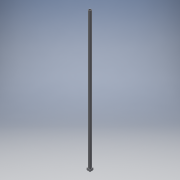
# Autodesk Inventor part: InnerLever
Saved by Autodesk Inventor 2017 (Build 210142000, 142)
## iProperties
Created: 2019-01-31
Part Number: InnerLever
Material: Generic
Document SubType Name: Modeling
Designer: S338674153
Density: 1 g/cm^3
Appearance: Default
Author: S338674153
Autodesk Inventor part; units mm, degrees
ref_plane "YZ Plane" through (0, 0, 0) normal (1, 0, 0) x (0, 1, 0)
ref_plane "XZ Plane" through (0, 0, 0) normal (0, 1, 0) x (-1, 0, 0)
ref_plane "XY Plane" through (0, 0, 0) normal (0, 0, 1) x (1, 0, 0)
sketch "Sketch1" plane through (0, 0, 0) normal (0, 1, 0) x (-1, 0, 0)
  circle A0 centre (0, 0) radius 6.985
  circle A1 centre (0, 0) radius 5.715
  dimension "d0" = 13.97
  dimension "d1" = 11.43
  constraints: 2 centre point, 2 coincident
  measures "d0" diameter of A0
  measures "d1" diameter of A1
extrude "Extrusion1" add sketch "Sketch1" along normal blind 660.4
sketch "Sketch3" plane through (0, 0, 0) normal (0, -1, 0) x (1, 0, 0)
  line L0 (7.62, -7.62) -> (-7.62, -7.62)
  line L1 (-7.62, -7.62) -> (-7.62, 7.62)
  line L2 (-7.62, 7.62) -> (7.62, 7.62)
  line L3 (7.62, 7.62) -> (7.62, -7.62)
  line L4 (7.62, 0) -> (-7.62, 0) construction
  line L5 (0, -7.62) -> (0, 7.62) construction
  point P0 (0, 0)
  point P1 (0, 0)
  dimension "d4" = 15.24
  dimension "d5" = 15.24
  dimension "d6" = 7.62
  dimension "d7" = 7.62
  constraints: 12 end point, 5 midpoint, 3 perpendicular, 2 parallel, 1 coincident, 1 horizontal
  measures "d4" distance of L2.end L0.start
  measures "d5" distance of L0.start L0.end
  measures "d6" distance between parallel lines of L0 L4
  measures "d7" distance between parallel lines of L5 L1
extrude "Extrusion2" add sketch "Sketch3" against normal blind 10.16 separate body
sketch "Sketch4" plane through (-7.62, 0, 7.62) normal (0, 0, 1) x (1, 0, 0)
  line L0 (0, 0) -> (0, 10.16) projected
  line L1 (15.24, 0) -> (15.24, 10.16) projected
  circle A0 centre (7.62, 5.08) radius 3.175
  point P0 (7.62, 0)
  dimension "d10" = 6.35
  constraints: 1 centre point
  measures "d10" diameter of A0
extrude "Extrusion3" cut sketch "Sketch4" against normal blind 26.3525 bodies 2
body "Solid1"
body "Solid2"
